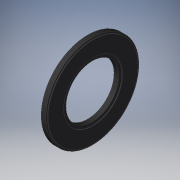
# Autodesk Inventor part: core_BA1730
Saved by Autodesk Inventor 2019 (Build 230136000, 136)
## iProperties
Created: 2023-09-05
Part Number: core_BA1730
Material: Generic
Catalog Web Link: www.cadenas.de
Description: BA_ _ _ _ __core-Thrust Needle Roller Bearings with Retainers
Vendor: MISUMI
Document SubType Name: Modeling
Designer: psAdmin
Manufacturer: MISUMI
Mass: 0.908313 g
Surface Area: 12.5664 cm^2
Volume: 0.908313 cm^3
Density: 1 g/cm^3
Appearance: PSOLRGB-175-175-175
Category: PARTsolutions
Company: MISUMI
Title: core_BA1730
Author: Cadenas PARTsolutions
Comments: Thrust Needle Roller Bearings with Retainers
PSOL_IDENT_0: {$CADENAS_DATA/23d-libs/misumi/metric/12_bearing_holders/core_ba1024.prj},172 {VTYP=3D},{NB=core_BA1
PSOL_IDENT_1: 730},{LINA=core_BA1730},{NN=BA_ _ _ _ __core},{DATE=19.10.2020 20:02:28},{GEOMDATE=19.10.2020 19:35:
PSOL_IDENT_2: 16},{VERSION=},{LINEID=40},{WBVAR=},{WBNUMERIC=}  {NB=core_BA1730},{LINA=core_BA1730},{KT=DUMMY},{TY
PSOL_IDENT_3: PE=BA1730},{DD=17},{D=30},{B=2},{F=29.0},{F1=19.0},{DD1=17},{D1=30},{B1=1}
NB: core_BA1730
NN: BA_ _ _ _ __core
NT: Thrust Needle Roller Bearings with Retainers
NBSYN: core_$TYPE.
LINA: core_BA1730
CATALOG: Misumi
TYPE: BA1730
DD: 17
D: 30
B: 2
F: 29
F1: 19
DD1: 17
D1: 30
B1: 1
SUPPLIER: MISUMI
ARTICLENO: core_BA1730
BOMINFO: core_BA1730
CREATOR: CADENAS GmbH
Autodesk Inventor part; units mm, degrees
sketch "Sketch_1" plane through (0, 0, 0) normal (0, 0, 1) x (1, 0, 0)
  line L0 (50, 0) -> (-50, 0)
  line L1 (-1, 9.5) -> (-0.75, 9.5)
  line L2 (-0.75, 9.5) -> (-0.75, 8.5)
  line L3 (-0.75, 8.5) -> (0.75, 8.5)
  line L4 (0.75, 8.5) -> (0.75, 9.5)
  line L5 (0.75, 9.5) -> (1, 9.5)
  line L6 (1, 9.5) -> (1, 14.5)
  line L7 (1, 14.5) -> (0.75, 14.5)
  line L8 (0.75, 14.5) -> (0.75, 15)
  line L9 (0.75, 15) -> (-0.75, 15)
  line L10 (-0.75, 15) -> (-0.75, 14.5)
  line L11 (-0.75, 14.5) -> (-1, 14.5)
  line L12 (-1, 14.5) -> (-1, 9.5)
  constraints: 26 end point
revolve "Revolution1" add sketch "Sketch_1" angle 360 about axis through (50, 0, 0) along (1, 0, 0)
ref_plane "core_to_washer_XY" through (0, 0, 0) normal (1, 0, 0) x (0, 0, -1)
ref_plane "core_to_washer_YZ" through (0, 0, 0) normal (0, 0, -1) x (0, 1, 0)
ref_plane "core_to_washer_ZX" through (0, 0, 0) normal (0, 1, 0) x (1, 0, 0)
ref_plane "core_to_washer1_XY" through (0, 0, 0) normal (-1, 0, 0) x (0, 0, -1)
ref_plane "core_to_washer1_YZ" through (0, 0, 0) normal (0, 0, -1) x (0, -1, 0)
ref_plane "core_to_washer1_ZX" through (0, 0, 0) normal (0, -1, 0) x (-1, 0, 0)
body "Solid1"
